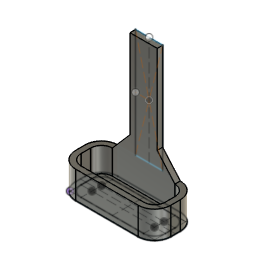
Power Bank Holder v8 (Autodesk Fusion 360 design; units mm, degrees)
Autodesk Fusion 360 part; units mm, degrees
sketch "Schizzo1" plane through (0, 0, 0) normal (0, 0, 1) x (1, 0, 0)
  line L0 (0, 0) -> (62, 0) construction
  line L1 (62, 0) -> (62, 23) construction
  line L2 (62, 23) -> (0, 23) construction
  line L3 (0, 23) -> (0, 0) construction
  line L4 (31, 23) -> (31, 0) construction
  line L5 (62, 23) -> (54, 23) construction
  line L6 (54, 23) -> (54, 0) construction
  line L7 (0, 23) -> (8, 23) construction
  line L8 (8, 23) -> (8, 0) construction
  line L9 (8, 0) -> (54, 0)
  line L10 (8, 23) -> (54, 23)
  line L11 (0, 23) -> (0, 15) construction
  line L12 (0, 15) -> (62, 15) construction
  line L13 (0, 0) -> (0, 8) construction
  line L14 (0, 8) -> (62, 8) construction
  line L15 (0, 15) -> (0, 8) construction
  line L16 (0, 15) -> (0, 8)
  line L17 (62, 15) -> (62, 8)
  arc A0 (8, 23) -> (0, 15) centre (8, 15) ccw
  arc A1 (0, 8) -> (8, 0) centre (8, 8) ccw
  arc A2 (54, 0) -> (62, 8) centre (54, 8) ccw
  arc A3 (62, 15) -> (54, 23) centre (54, 15) ccw
  arc A4 (66, 15) -> (54, 27) centre (54, 15) ccw
  line L18 (8, 27) -> (54, 27)
  arc A5 (8, 27) -> (-4, 15) centre (8, 15) ccw
  line L19 (-4, 15) -> (-4, 8)
  arc A6 (-4, 8) -> (8, -4) centre (8, 8) ccw
  line L20 (8, -4) -> (54, -4)
  arc A7 (54, -4) -> (66, 8) centre (54, 8) ccw
  line L21 (66, 15) -> (66, 8)
  line L22 (0, 11.5) -> (62, 11.5) construction
  line L23 (0, 11.5) -> (-4, 11.5) construction
  line L24 (62, 11.5) -> (66, 11.5) construction
  dimension "d10" = 62
  dimension "d11" = 23
  dimension "d12" = 8
  dimension "d13" = 8
  dimension "d15" = 8
  dimension "d16" = 8
  dimension "d17" = -4
  dimension "d32" = 70
  dimension "d33" = 31
  constraint horizontal L0
  constraint vertical L1
  constraint horizontal L2
  constraint vertical L3
  constraint coincident L0.start L3.end
  constraint midpoint L2 L4.start
  constraint midpoint L0 L4.end
  constraint perpendicular L1 L5
  constraint coincident L0 L6.end
  constraint perpendicular L0 L6
  constraint perpendicular L3 L7
  constraint coincident L0 L8.end
  constraint perpendicular L0 L8
  constraint perpendicular L2 L11
  constraint coincident L1 L12.end
  constraint perpendicular L1 L12
  constraint perpendicular L0 L13
  constraint coincident L1 L14.end
  constraint perpendicular L1 L14
  constraint tangent L15 A0
  constraint tangent L15 A1
  constraint tangent L9 A2
  constraint tangent L17 A3
  constraint midpoint L15 L22.start
  constraint midpoint L17 L22.end
  constraint perpendicular L19 L23
  constraint perpendicular L21 L24
  constraint coincident L19 L23.end
  constraint coincident L21 L24.end
  measures "d10" distance of L0.start L0.end
  measures "d11" distance of L0.start L2.end
  measures "d12" distance of L1.end L5.end
  measures "d13" distance of L2.end L7.end
  measures "d15" distance of L2.end L11.end
  measures "d16" distance of L0.start L13.end
  measures "d32" distance of L19 L21
  measures "d33" distance of L18 L20
extrude "Estrusione2" add sketch "Schizzo1" along normal blind 20
extrude "Estrusione4" add sketch "Schizzo1" along normal blind 2 contours L9 L10 L16 L17 A0 A1 A2 A3
sketch "Schizzo3" plane through (0, 27, 0) normal (0, 1, 0) x (-1, 0, 0)
  line L0 (-54, 0) -> (-8, 0)
  line L1 (-8, 0) -> (-8, 20)
  line L2 (-8, 20) -> (-54, 20)
  line L3 (-54, 20) -> (-54, 0)
  line L4 (-31, 20) -> (-31, 100) construction
  line L5 (-31, 60) -> (-21, 60) construction
  line L6 (-21, 20) -> (-41, 20)
  line L7 (-41, 20) -> (-41, 100)
  line L8 (-41, 100) -> (-21, 100)
  line L9 (-21, 100) -> (-21, 20)
  line L10 (-21, 20) -> (-41, 100) construction
  line L11 (-41, 20) -> (-21, 100) construction
  point P0 (-31, 60)
  dimension "d22" = 20
  dimension "d23" = 80
  constraint midpoint L2 L4.start
  constraint perpendicular L2 L4
  constraint midpoint L4 P0
  constraint perpendicular L4 L5
  constraint horizontal L6
  constraint perpendicular L6 L7
  constraint parallel L6 L8
  constraint parallel L7 L9
  constraint coincident L10 P0
  constraint coincident L11 P0
  constraint coincident P0 L5.start
  measures "d22" distance of L7.end L8.end
  measures "d23" distance of L6.end L7.end
extrude "Estrusione3" add sketch "Schizzo3" against normal blind 4 contours L2 L6 L7 L8 L9
sketch "Schizzo4" plane through (0, 27, 0) normal (0, 1, 0) x (-1, 0, 0)
  line L0 (-54, 0) -> (-8, 0)
  line L1 (-8, 0) -> (-8, 20)
  line L2 (-8, 20) -> (-21, 20)
  line L3 (-21, 20) -> (-21, 100)
  line L4 (-21, 100) -> (-41, 100)
  line L5 (-41, 100) -> (-41, 20)
  line L6 (-41, 20) -> (-54, 20)
  line L7 (-54, 20) -> (-54, 0)
  line L8 (-54, 20) -> (-41, 35)
  line L9 (-31, 100) -> (-31, -12.8301) construction
  line L10 (-8, 20) -> (-21, 35)
  constraint coincident L6.end L7.start
  constraint coincident L5 L8.end
  constraint midpoint L4 L9.start
  constraint perpendicular L0 L9
  constraint symmetric L6.end L9 L1.end
  constraint symmetric L8.end L9 L10.end
extrude "Estrusione5" add sketch "Schizzo4" against normal blind 4 contours L5 L6 L8 | L2 L3 L10
equation "d12 = d13"
equation "d15 = d13"
equation "d16 = d13"
